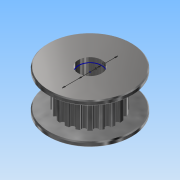
# Autodesk Inventor part: Шкив 2GT с подшипником 5мм
Saved by Autodesk Inventor 2017 (Build 210142000, 142)
## iProperties
Part Number: Шкив 2GT с подшипником 5мм
Material: Типовые
Document SubType Name: Modeling
Designer: STALKER
Density: 1 g/cm^3
Appearance: Сталь - гальванизированная
Mass: 1.02016 g
Surface Area: 13.4398 cm^2
Volume: 1.02016 cm^3
Author: STALKER
Autodesk Inventor part; units mm, degrees
ref_plane "YZ Plane" through (0, 0, 0) normal (1, 0, 0) x (0, 1, 0)
ref_plane "XZ Plane" through (0, 0, 0) normal (0, 1, 0) x (-1, 0, 0)
ref_plane "XY Plane" through (0, 0, 0) normal (0, 0, 1) x (1, 0, 0)
sketch "Эскиз1" plane through (0, 0, 0) normal (0, 0, 1) x (1, 0, 0)
  line L0 (0, 0) -> (-6.1125, 0) construction
  line L1 (0, 0) -> (0, 16.0328) construction
  circle A0 centre (0, 0) radius 5.8625 construction
  arc A1 (-0.4857, 5.7438) -> (0.4857, 5.7438) centre (0, 5.8625) ccw
  line L2 (-0.5277, 5.9157) -> (-0.4857, 5.7438)
  line L3 (0.5277, 5.9157) -> (0.4857, 5.7438)
  arc A2 (0.7464, 6.0668) -> (0.5277, 5.9157) centre (0.722, 5.8683) ccw
  arc A3 (-0.5277, 5.9157) -> (-0.7464, 6.0668) centre (-0.722, 5.8683) ccw
  arc A4 (-2.2369, 5.3126) -> (-1.313, 5.6128) centre (-1.8116, 5.5756) ccw
  line L4 (-2.3299, 5.4631) -> (-2.2369, 5.3126)
  line L5 (-1.3262, 5.7893) -> (-1.313, 5.6128)
  arc A5 (-1.1648, 6.0005) -> (-1.3262, 5.7893) centre (-1.1267, 5.8041) ccw
  arc A6 (-2.3299, 5.4631) -> (-2.5846, 5.5392) centre (-2.5001, 5.3579) ccw
  arc A7 (-3.7691, 4.3614) -> (-2.9832, 4.9323) centre (-3.4459, 4.7429) ccw
  line L6 (-3.9041, 4.4757) -> (-3.7691, 4.3614)
  line L7 (-3.0502, 5.0961) -> (-2.9832, 4.9323)
  arc A8 (-2.9621, 5.3468) -> (-3.0502, 5.0961) centre (-2.8652, 5.1719) ccw
  arc A9 (-3.9041, 4.4757) -> (-4.1698, 4.4694) centre (-4.0334, 4.3231) ccw
  arc A10 (-4.9323, 2.9832) -> (-4.3614, 3.7691) centre (-4.7429, 3.4459) ccw
  line L8 (-5.0961, 3.0502) -> (-4.9323, 2.9832)
  line L9 (-4.4757, 3.9041) -> (-4.3614, 3.7691)
  arc A11 (-4.4694, 4.1698) -> (-4.4757, 3.9041) centre (-4.3231, 4.0334) ccw
  arc A12 (-5.0961, 3.0502) -> (-5.3468, 2.9621) centre (-5.1719, 2.8652) ccw
  arc A13 (-5.6128, 1.313) -> (-5.3126, 2.2369) centre (-5.5756, 1.8116) ccw
  line L10 (-5.7893, 1.3262) -> (-5.6128, 1.313)
  line L11 (-5.4631, 2.3299) -> (-5.3126, 2.2369)
  arc A14 (-5.5392, 2.5846) -> (-5.4631, 2.3299) centre (-5.3579, 2.5001) ccw
  arc A15 (-5.7893, 1.3262) -> (-6.0005, 1.1648) centre (-5.8041, 1.1267) ccw
  arc A16 (-5.7438, -0.4857) -> (-5.7438, 0.4857) centre (-5.8625, 0) ccw
  line L12 (-5.9157, -0.5277) -> (-5.7438, -0.4857)
  line L13 (-5.9157, 0.5277) -> (-5.7438, 0.4857)
  arc A17 (-6.0668, 0.7464) -> (-5.9157, 0.5277) centre (-5.8683, 0.722) ccw
  arc A18 (-5.9157, -0.5277) -> (-6.0668, -0.7464) centre (-5.8683, -0.722) ccw
  arc A19 (-5.3126, -2.2369) -> (-5.6128, -1.313) centre (-5.5756, -1.8116) ccw
  line L14 (-5.4631, -2.3299) -> (-5.3126, -2.2369)
  line L15 (-5.7893, -1.3262) -> (-5.6128, -1.313)
  arc A20 (-6.0005, -1.1648) -> (-5.7893, -1.3262) centre (-5.8041, -1.1267) ccw
  arc A21 (-5.4631, -2.3299) -> (-5.5392, -2.5846) centre (-5.3579, -2.5001) ccw
  arc A22 (-4.3614, -3.7691) -> (-4.9323, -2.9832) centre (-4.7429, -3.4459) ccw
  line L16 (-4.4757, -3.9041) -> (-4.3614, -3.7691)
  line L17 (-5.0961, -3.0502) -> (-4.9323, -2.9832)
  arc A23 (-5.3468, -2.9621) -> (-5.0961, -3.0502) centre (-5.1719, -2.8652) ccw
  arc A24 (-4.4757, -3.9041) -> (-4.4694, -4.1698) centre (-4.3231, -4.0334) ccw
  arc A25 (-2.9832, -4.9323) -> (-3.7691, -4.3614) centre (-3.4459, -4.7429) ccw
  line L18 (-3.0502, -5.0961) -> (-2.9832, -4.9323)
  line L19 (-3.9041, -4.4757) -> (-3.7691, -4.3614)
  arc A26 (-4.1698, -4.4694) -> (-3.9041, -4.4757) centre (-4.0334, -4.3231) ccw
  arc A27 (-3.0502, -5.0961) -> (-2.9621, -5.3468) centre (-2.8652, -5.1719) ccw
  arc A28 (-1.313, -5.6128) -> (-2.2369, -5.3126) centre (-1.8116, -5.5756) ccw
  line L20 (-1.3262, -5.7893) -> (-1.313, -5.6128)
  line L21 (-2.3299, -5.4631) -> (-2.2369, -5.3126)
  arc A29 (-2.5846, -5.5392) -> (-2.3299, -5.4631) centre (-2.5001, -5.3579) ccw
  arc A30 (-1.3262, -5.7893) -> (-1.1648, -6.0005) centre (-1.1267, -5.8041) ccw
  arc A31 (0.4857, -5.7438) -> (-0.4857, -5.7438) centre (0, -5.8625) ccw
  line L22 (0.5277, -5.9157) -> (0.4857, -5.7438)
  line L23 (-0.5277, -5.9157) -> (-0.4857, -5.7438)
  arc A32 (-0.7464, -6.0668) -> (-0.5277, -5.9157) centre (-0.722, -5.8683) ccw
  arc A33 (0.5277, -5.9157) -> (0.7464, -6.0668) centre (0.722, -5.8683) ccw
  arc A34 (2.2369, -5.3126) -> (1.313, -5.6128) centre (1.8116, -5.5756) ccw
  line L24 (2.3299, -5.4631) -> (2.2369, -5.3126)
  line L25 (1.3262, -5.7893) -> (1.313, -5.6128)
  arc A35 (1.1648, -6.0005) -> (1.3262, -5.7893) centre (1.1267, -5.8041) ccw
  arc A36 (2.3299, -5.4631) -> (2.5846, -5.5392) centre (2.5001, -5.3579) ccw
  arc A37 (3.7691, -4.3614) -> (2.9832, -4.9323) centre (3.4459, -4.7429) ccw
  line L26 (3.9041, -4.4757) -> (3.7691, -4.3614)
  line L27 (3.0502, -5.0961) -> (2.9832, -4.9323)
  arc A38 (2.9621, -5.3468) -> (3.0502, -5.0961) centre (2.8652, -5.1719) ccw
  arc A39 (3.9041, -4.4757) -> (4.1698, -4.4694) centre (4.0334, -4.3231) ccw
  arc A40 (4.9323, -2.9832) -> (4.3614, -3.7691) centre (4.7429, -3.4459) ccw
  line L28 (5.0961, -3.0502) -> (4.9323, -2.9832)
  line L29 (4.4757, -3.9041) -> (4.3614, -3.7691)
  arc A41 (4.4694, -4.1698) -> (4.4757, -3.9041) centre (4.3231, -4.0334) ccw
  arc A42 (5.0961, -3.0502) -> (5.3468, -2.9621) centre (5.1719, -2.8652) ccw
  arc A43 (5.6128, -1.313) -> (5.3126, -2.2369) centre (5.5756, -1.8116) ccw
  line L30 (5.7893, -1.3262) -> (5.6128, -1.313)
  line L31 (5.4631, -2.3299) -> (5.3126, -2.2369)
  arc A44 (5.5392, -2.5846) -> (5.4631, -2.3299) centre (5.3579, -2.5001) ccw
  arc A45 (5.7893, -1.3262) -> (6.0005, -1.1648) centre (5.8041, -1.1267) ccw
  arc A46 (5.7438, 0.4857) -> (5.7438, -0.4857) centre (5.8625, 0) ccw
  line L32 (5.9157, 0.5277) -> (5.7438, 0.4857)
  line L33 (5.9157, -0.5277) -> (5.7438, -0.4857)
  arc A47 (6.0668, -0.7464) -> (5.9157, -0.5277) centre (5.8683, -0.722) ccw
  arc A48 (5.9157, 0.5277) -> (6.0668, 0.7464) centre (5.8683, 0.722) ccw
  arc A49 (5.3126, 2.2369) -> (5.6128, 1.313) centre (5.5756, 1.8116) ccw
  line L34 (5.4631, 2.3299) -> (5.3126, 2.2369)
  line L35 (5.7893, 1.3262) -> (5.6128, 1.313)
  arc A50 (6.0005, 1.1648) -> (5.7893, 1.3262) centre (5.8041, 1.1267) ccw
  arc A51 (5.4631, 2.3299) -> (5.5392, 2.5846) centre (5.3579, 2.5001) ccw
  arc A52 (4.3614, 3.7691) -> (4.9323, 2.9832) centre (4.7429, 3.4459) ccw
  line L36 (4.4757, 3.9041) -> (4.3614, 3.7691)
  line L37 (5.0961, 3.0502) -> (4.9323, 2.9832)
  arc A53 (5.3468, 2.9621) -> (5.0961, 3.0502) centre (5.1719, 2.8652) ccw
  arc A54 (4.4757, 3.9041) -> (4.4694, 4.1698) centre (4.3231, 4.0334) ccw
  arc A55 (2.9832, 4.9323) -> (3.7691, 4.3614) centre (3.4459, 4.7429) ccw
  line L38 (3.0502, 5.0961) -> (2.9832, 4.9323)
  line L39 (3.9041, 4.4757) -> (3.7691, 4.3614)
  arc A56 (4.1698, 4.4694) -> (3.9041, 4.4757) centre (4.0334, 4.3231) ccw
  arc A57 (3.0502, 5.0961) -> (2.9621, 5.3468) centre (2.8652, 5.1719) ccw
  arc A58 (1.313, 5.6128) -> (2.2369, 5.3126) centre (1.8116, 5.5756) ccw
  line L40 (1.3262, 5.7893) -> (1.313, 5.6128)
  line L41 (2.3299, 5.4631) -> (2.2369, 5.3126)
  arc A59 (2.5846, 5.5392) -> (2.3299, 5.4631) centre (2.5001, 5.3579) ccw
  arc A60 (1.3262, 5.7893) -> (1.1648, 6.0005) centre (1.1267, 5.8041) ccw
  arc A61 (1.1648, 6.0005) -> (0.7464, 6.0668) centre (0, 0) ccw
  arc A62 (2.9621, 5.3468) -> (2.5846, 5.5392) centre (0, 0) ccw
  arc A63 (4.4694, 4.1698) -> (4.1698, 4.4694) centre (0, 0) ccw
  arc A64 (5.5392, 2.5846) -> (5.3468, 2.9621) centre (0, 0) ccw
  arc A65 (6.0668, 0.7464) -> (6.0005, 1.1648) centre (0, 0) ccw
  arc A66 (6.0005, -1.1648) -> (6.0668, -0.7464) centre (0, 0) ccw
  arc A67 (5.3468, -2.9621) -> (5.5392, -2.5846) centre (0, 0) ccw
  arc A68 (4.1698, -4.4694) -> (4.4694, -4.1698) centre (0, 0) ccw
  arc A69 (2.5846, -5.5392) -> (2.9621, -5.3468) centre (0, 0) ccw
  arc A70 (0.7464, -6.0668) -> (1.1648, -6.0005) centre (0, 0) ccw
  arc A71 (-1.1648, -6.0005) -> (-0.7464, -6.0668) centre (0, 0) ccw
  arc A72 (-2.9621, -5.3468) -> (-2.5846, -5.5392) centre (0, 0) ccw
  arc A73 (-4.4694, -4.1698) -> (-4.1698, -4.4694) centre (0, 0) ccw
  arc A74 (-5.5392, -2.5846) -> (-5.3468, -2.9621) centre (0, 0) ccw
  arc A75 (-6.0668, -0.7464) -> (-6.0005, -1.1648) centre (0, 0) ccw
  arc A76 (-6.0005, 1.1648) -> (-6.0668, 0.7464) centre (0, 0) ccw
  arc A77 (-5.3468, 2.9621) -> (-5.5392, 2.5846) centre (0, 0) ccw
  arc A78 (-4.1698, 4.4694) -> (-4.4694, 4.1698) centre (0, 0) ccw
  arc A79 (-0.7464, 6.0668) -> (-1.1648, 6.0005) centre (0, 0) ccw
  arc A80 (-2.5846, 5.5392) -> (-2.9621, 5.3468) centre (0, 0) ccw
  circle A81 centre (0, 0) radius 5
  circle A82 centre (0, 0) radius 9
  circle A83 centre (0, 0) radius 2.5
  circle A84 centre (0, 0) radius 4.6
  circle A85 centre (0, 0) radius 2.9
  point P0 (-0.5693, 6.0859)
  point P1 (0.5693, 6.0859)
  point P2 (-2.4221, 5.6121)
  point P3 (-1.3392, 5.964)
  point P4 (-4.0378, 4.589)
  point P5 (-3.1166, 5.2583)
  point P6 (-5.2583, 3.1166)
  point P7 (-4.589, 4.0378)
  point P8 (-5.964, 1.3392)
  point P9 (-5.6121, 2.4221)
  point P10 (-6.0859, -0.5693)
  point P11 (-6.0859, 0.5693)
  point P12 (-5.6121, -2.4221)
  point P13 (-5.964, -1.3392)
  point P14 (-4.589, -4.0378)
  point P15 (-5.2583, -3.1166)
  point P16 (-3.1166, -5.2583)
  point P17 (-4.0378, -4.589)
  point P18 (-1.3392, -5.964)
  point P19 (-2.4221, -5.6121)
  point P20 (0.5693, -6.0859)
  point P21 (-0.5693, -6.0859)
  point P22 (2.4221, -5.6121)
  point P23 (1.3392, -5.964)
  point P24 (4.0378, -4.589)
  point P25 (3.1166, -5.2583)
  point P26 (5.2583, -3.1166)
  point P27 (4.589, -4.0378)
  point P28 (5.964, -1.3392)
  point P29 (5.6121, -2.4221)
  point P30 (6.0859, 0.5693)
  point P31 (6.0859, -0.5693)
  point P32 (5.6121, 2.4221)
  point P33 (5.964, 1.3392)
  point P34 (4.589, 4.0378)
  point P35 (5.2583, 3.1166)
  point P36 (3.1166, 5.2583)
  point P37 (4.0378, 4.589)
  point P38 (1.3392, 5.964)
  point P39 (2.4221, 5.6121)
  dimension "d1" = 11.725
  dimension "d2" = 1
  dimension "d4" = 0.2
  dimension "d5" = 0.2
  dimension "d8" = 360
  dimension "d10" = 10
  dimension "d11" = 18
  dimension "d12" = 5
  dimension "d13" = 0.4
  dimension "d14" = 0.4
  constraints: 160 point on circle, 86 centre point, 84 end point, 41 point on line, 7 coincident, 4 tangent, 1 horizontal, 1 vertical, 321 other
  measures "d1" diameter of A0
  measures "d2" diameter of A1
  measures "d4" radius of A2
  measures "d5" radius of A3
  measures "d10" diameter of A81
  measures "d11" diameter of A82
  measures "d12" diameter of A83
  measures "d13" radial gap between concentric circles of A81 A84
  measures "d14" radial gap between concentric circles of A85 A83
extrude "Выдавливание1" add sketch "Эскиз1" along normal mid plane 8.7 contours A1 L3 A2 A61 A60 L40 A58 L41 A59 A62 A57 L38 A55 L39 A56 A63 A54 L36 A52 L37 A53 A64 A51 L34 A49 L35 A50 A65 A48 L32 A46 L33 A47 A66 A45 L30 A43 L31 A44 A67 A42 L28 A40 L29 A41 A68 A39 L26 A37 L27 A38 A69 A36 L24 A34 L25 A35 A70 A33 L22 A31 L23 A32 A71 A30 L20 A28 L21 A29 A72 A27 L18 A25 L19 A26 A73 A24 L16 A22 L17 A23 A74 A21 L14 A19 L15 A20 A75 A18 L12 A16 L13 A17 A76 A15 L10 A13 L11 A14 A77 A12 L8 A10 L9 A11 A78 A9 L6 A7 L7 A8 A80 A6 L4 A4 L5 A5 A79 A3 L2 | A82
extrude "Выдавливание2" cut sketch "Эскиз1" along normal mid plane 6.7 contours A82
extrude "Выдавливание3" add sketch "Эскиз1" along normal mid plane 8.7 contours A81 | A85
extrude "Выдавливание4" add sketch "Эскиз1" along normal mid plane 8.7 contours A84
chamfer "Фаска2" distance 0.2 angle 45 4 edges at (-9, 0, 4.35) (-9, 0, 3.35) (-9, 0, -3.35) (-9, 0, -4.35)
sketch "Эскиз2" plane through (0, 0, 3.35) normal (0, 0, -1) x (-1, 0, 0)
  circle A0 centre (0, 0) radius 6
  circle A1 centre (0, 0) radius 2.5
  circle A2 centre (0, 0) radius 7.5981
  dimension "d29" = 12
  dimension "d30" = 5
  constraints: 3 centre point, 3 coincident
  measures "d29" diameter of A0
  measures "d30" diameter of A1
extrude "Выдавливание5" cut sketch "Эскиз2" along normal blind 6.7 contours A2
